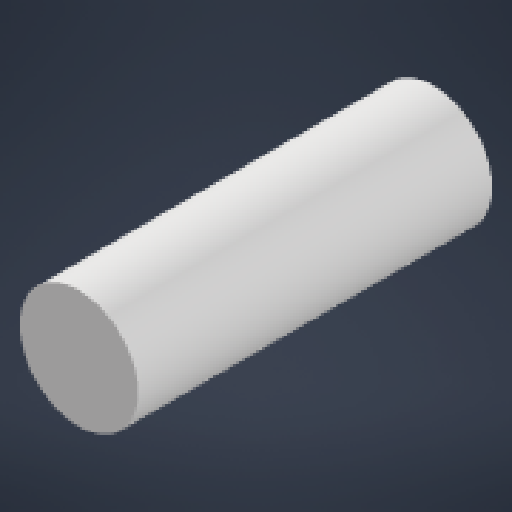
# Autodesk Inventor part: base worm
Saved by Autodesk Inventor 2024 (Build 280153000, 153)
## iProperties
Created: 2023-06-18
Part Number: base worm
Material: 일반
Document SubType Name: Modeling
Designer: 6gioc
Density: 1 g/cm^3
Appearance: 기본값
Author: 6gioc
Autodesk Inventor part; units mm, degrees
ref_plane "YZ Plane" through (0, 0, 0) normal (1, 0, 0) x (0, 1, 0)
ref_plane "XZ Plane" through (0, 0, 0) normal (0, 1, 0) x (-1, 0, 0)
ref_plane "XY Plane" through (0, 0, 0) normal (0, 0, 1) x (1, 0, 0)
sketch "스케치1" plane through (0, 0, 0) normal (0, 0, 1) x (1, 0, 0)
  circle A0 centre (0, 0) radius 5
  circle A1 centre (0, 0) radius 2.5
  line L0 (2.5, 0) -> (-2, 0)
  line L1 (-2, 0) -> (-2, 1.5)
  line L2 (-2, 0) -> (-2, -1.5)
  dimension "d0" = 10
  dimension "d1" = 5
  dimension "d2" = 4.5
  constraints: 6 end point, 3 point on circle, 2 centre point, 2 coincident, 1 horizontal, 1 perpendicular, 1 point on line
  measures "d0" diameter of A0
  measures "d1" diameter of A1
  measures "d2" distance of L0.start L0.end
extrude "돌출1" add sketch "스케치1" against normal blind 15 contours A0 | L1 L2 A1
extrude "돌출2" add sketch "스케치1" along normal blind 15 contours A0 | L0 L1 A1 | A1 L2 L0 | L1 L2 A1
